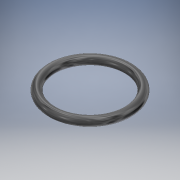
# Autodesk Inventor part: Oring3_3
Saved by Autodesk Inventor 2018 (Build 220112000, 112)
## iProperties
Shininess: 64.0
Length Units: 11269
Angle Units: 11279
Time Units: 11290
Mass Units: 11283
Length Display Precision: 3
Angle Display Precision: 2
Created: 2002-03-02
Part Number: Oring3_3
Document SubType Name: Modeling
Designer: Default
Material: Silicone
Density: 1.25 g/cm^3
Appearance: Rubber - Black - Version 1.1
Density: 0.0
Volumn: 0.0
Area: 0.0
PropertySet Name: Model Information
Control State: 0
Master: False
Checked Out: False
Author: Default
Autodesk Inventor part; units mm, degrees
ref_plane "YZ Plane" through (0, 0, 0) normal (1, 0, 0) x (0, 1, 0)
ref_plane "XZ Plane" through (0, 0, 0) normal (0, 1, 0) x (-1, 0, 0)
ref_plane "XY Plane" through (0, 0, 0) normal (0, 0, 1) x (1, 0, 0)
sketch "Sketch2" plane through (0, 0, 0) normal (0, 1, 0) x (-1, 0, 0)
  line L0 (1, 0) -> (-13, 0) projected
  line L1 (0, -1.2) -> (0, 1.6) projected
  circle A0 centre (-9, 0) radius 1
  point P0 (0, 0)
  dimension "d0" = 2
  dimension "d1" = 18
  constraints: 1 centre point, 1 point on line
  measures "d0" diameter of A0
  measures "d1" diameter of A0.centre L1
revolve "Revolution1" add sketch "Sketch2" angle 360 about axis through (0, 0, -10) along (0, 0, 1)
body "Solid1"
